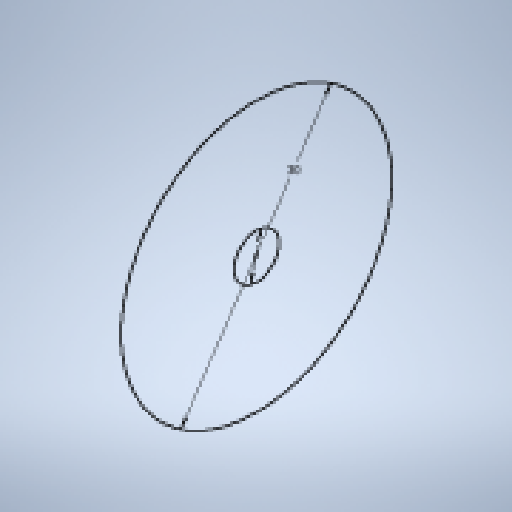
# Autodesk Inventor part: Arm_2
Saved by Autodesk Inventor 2023 (Build 270158000, 158)
## iProperties
Created: 2022-04-08
Part Number: Arm_2
Material: 一般
Document SubType Name: Modeling
Designer: device
Density: 1 g/cm^3
Appearance: 預設
Author: device
Autodesk Inventor part; units mm, degrees
ref_plane "YZ Plane" through (0, 0, 0) normal (1, 0, 0) x (0, 1, 0)
ref_plane "XZ Plane" through (0, 0, 0) normal (0, 1, 0) x (-1, 0, 0)
ref_plane "XY Plane" through (0, 0, 0) normal (0, 0, 1) x (1, 0, 0)
sketch "草圖1" plane through (0, 0, 0) normal (1, 0, 0) x (0, 1, 0)
  circle A0 centre (0, 0) radius 2.5
  circle A1 centre (0, 0) radius 15
  dimension "d0" = 5
  dimension "d1" = 30
  constraints: 2 centre point, 2 coincident
  measures "d0" diameter of A0
  measures "d1" diameter of A1
extrude "擠出1" add sketch "草圖1" along normal mid plane 3
sketch "草圖2" plane through (1.5, 0, 0) normal (1, 0, 0) x (0, 0, -1)
  line L0 (-9.5551, 8.1555) -> (8.9449, 8.1555)
  line L1 (8.9449, 8.1555) -> (8.9449, 5.1555)
  line L2 (8.9449, 5.1555) -> (-9.5551, 5.1555)
  line L3 (-9.5551, 5.1555) -> (-9.5551, 8.1555)
  point P0 (0, 0)
  dimension "d4" = 18.5
  dimension "d5" = 3
  constraints: 8 end point, 2 parallel, 1 perpendicular
  measures "d4" distance of L0.start L0.end
  measures "d5" distance of L2.end L0.start
extrude "擠出2" add sketch "草圖2" along normal blind 47
sketch "草圖3" plane through (1.5, 8.1555, 9.5551) normal (0, 1, 0) x (1, 0, 0)
  line L0 (0, 18.5) -> (47, 18.5) construction
  line L1 (41, 18.5) -> (17, 18.5)
  line L2 (17, 18.5) -> (17, 6)
  line L3 (17, 6) -> (41, 6)
  line L4 (41, 6) -> (41, 18.5)
  line L5 (47, 18.5) -> (47, 0) construction
  line L6 (47, 0) -> (47, 18.5) projected
  line L7 (47, 12.25) -> (14.3759, 12.25) construction
  circle A0 centre (43.5, 12.25) radius 1.25
  line L8 (29, 12.25) -> (29, 6) construction
  circle A1 centre (14.5, 12.25) radius 1.25
  point P0 (-1.5, 9.5551)
  point P1 (41, 12.25)
  dimension "d8" = 24
  dimension "d9" = 12.5
  dimension "d10" = 6
  dimension "d11" = 2.5
  dimension "d12" = 29
  constraints: 12 end point, 6 point on line, 2 centre point, 2 midpoint, 2 parallel, 2 perpendicular, 1 horizontal, 1 symmetric about line, 1 other
  measures "d8" distance of L2.end L3.end
  measures "d9" distance of L1.end L2.end
  measures "d10" distance between parallel lines of L5 L4
  measures "d11" diameter of A0
  measures "d12" distance of A1.centre A0.centre
extrude "擠出3" cut sketch "草圖3" against normal up to surface (3 mm away)
sketch "草圖4" plane through (1.5, 0, 0) normal (1, 0, 0) x (0, 0, -1)
  line L0 (-9.5551, 8.1555) -> (8.9449, 8.1555) projected
  line L1 (-12.5892, 8.1555) -> (12.5892, 8.1555)
  circle A0 centre (0, 0) radius 15 projected
  constraints: 2 end point, 2 point on circle, 1 collinear, 1 horizontal
extrude "擠出4" cut sketch "草圖4" against normal up to surface (3 mm away) contours L1 A0 L0 picked at (-0.2034, 10.437)
